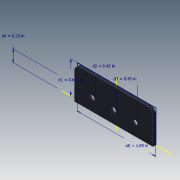
# Autodesk Inventor part: FL UPSTOP FLAP
Saved by Autodesk Inventor 2020.3 (Build 243373000, 373)
## iProperties
RuleStatus: InUse
AfterDocSave0: file://Part Number Cleaner
Created: 2020-02-12
Material: DELRIN 100, BLACK (EXTRUDED)
Vendor: HHMI: JRC - ID&F
Document SubType Name: Modeling
Designer: arnoldj
Density: 1.42 g/cm^3
Appearance: Black Anodize
DESIGN DEPARTMENT: HHMI: JRC - ID&F
ALTERED ITEM PART NUMBER: N/A
ALTERED ITEM VENDOR: N/A
ALTERED ITEM DESCRIPTION: N/A
Author: arnoldj
Revision Number: 0
Autodesk Inventor part; units mm, degrees
ref_plane "YZ Plane" through (0, 0, 0) normal (1, 0, 0) x (0, 1, 0)
ref_plane "XZ Plane" through (0, 0, 0) normal (0, 1, 0) x (-1, 0, 0)
ref_plane "XY Plane" through (0, 0, 0) normal (0, 0, 1) x (1, 0, 0)
sketch "Sketch1" plane through (0, 0, 0) normal (0, 0, 1) x (1, 0, 0)
  line L0 (0, 20.574) -> (0, -3.429) projected
  line L1 (-29.337, 0) -> (29.337, 0) projected
  line L2 (20.955, 17.145) -> (-20.955, 17.145)
  line L3 (-20.955, 17.145) -> (-20.955, 0)
  line L4 (-20.955, 0) -> (20.955, 0)
  line L5 (20.955, 0) -> (20.955, 17.145)
  line L6 (20.955, 17.145) -> (-20.955, 0) construction
  line L7 (-20.955, 17.145) -> (20.955, 0) construction
  point P0 (0, 0)
  point P1 (0, 8.5725)
  point P2 (-11.43, 6.35)
  point P3 (0, 6.35)
  point P4 (11.43, 6.35)
  dimension "d0" = 41.91
  dimension "d1" = 17.145
  dimension "d2" = 11.43
  dimension "d3" = 11.43
  dimension "d4" = 6.35
  constraints: 12 end point, 3 midpoint, 2 horizontal alignment, 2 parallel, 2 point on line, 1 horizontal, 1 perpendicular
  measures "d0" distance between parallel lines of L5 L3
  measures "d1" distance of L2.end L3.end
  measures "d2" distance of point (0, 6.35) point (-11.43, 6.35)
  measures "d3" distance of point (0, 6.35) point (11.43, 6.35)
  measures "d4" distance from line of point (-11.43, 6.35) L1
extrude "Extrusion1" add sketch "Sketch1" along normal blind 1.524
fillet "Fillet1" radius 3.175 2 edges at (20.955, 17.145, 0.762) (-20.955, 17.145, 0.762)
hole "Hole1" at (-11.43, 6.35, 0) at (0, 6.35, 0) at (11.43, 6.35, 0) direction (0, 0, 1) diameter 2.4384 end through all countersink diameter 4.3688 countersink angle 82 clearance for "Flat Head Machine Screw (82)" size "#2" standard "Ansi Unified Screw Threads"
body "Solid1"
